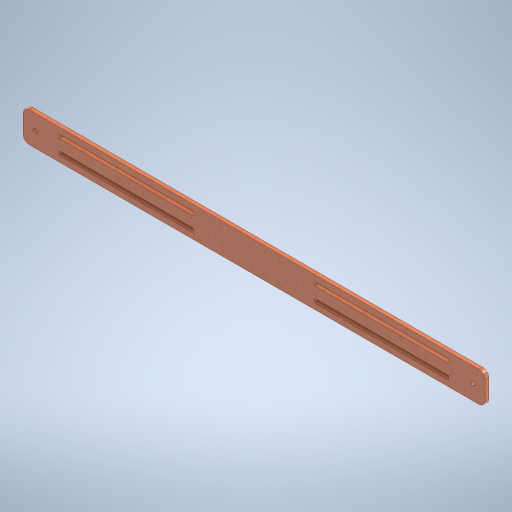
# Autodesk Inventor part: Pared
Saved by Autodesk Inventor 2024 (Build 280153000, 153)
## iProperties
Created: 2023-11-01
Part Number: Pared
Material: Generic
Document SubType Name: Modeling
Designer: fredy
Density: 1 g/cm^3
Appearance: Walnut - Natural Polished
Author: fredy
Autodesk Inventor part; units mm, degrees
ref_plane "YZ Plane" through (0, 0, 0) normal (1, 0, 0) x (0, 1, 0)
ref_plane "XZ Plane" through (0, 0, 0) normal (0, 1, 0) x (-1, 0, 0)
ref_plane "XY Plane" through (0, 0, 0) normal (0, 0, 1) x (1, 0, 0)
sketch "Sketch1" plane through (0, 0, 0) normal (0, 0, 1) x (1, 0, 0)
  line L0 (0, 0) -> (380, 0)
  line L1 (0, 0) -> (0, 25)
  line L2 (0, 25) -> (380, 25)
  line L3 (380, 25) -> (380, 0)
  dimension "d0" = 380
  dimension "d1" = 25
  constraints: 8 end point, 2 horizontal, 2 vertical, 1 coincident
  measures "d0" distance of L1.end L2.end
  measures "d1" distance of L0.start L1.end
extrude "Extrusion1" add sketch "Sketch1" along normal blind 3
fillet "Fillet1" radius 5 4 edges at (380, 25, 1.5) (380, 0, 1.5) (0, 25, 1.5) (0, 0, 1.5)
sketch "Sketch2" plane through (0, 0, 3) normal (0, 0, 1) x (1, 0, 0)
  line L0 (30, 16.9) -> (140, 16.9)
  line L1 (140, 16.9) -> (140, 20)
  line L2 (140, 20) -> (30, 20)
  line L3 (30, 20) -> (30, 16.9)
  line L4 (375, 25) -> (5, 25) projected
  line L5 (0, 20) -> (0, 5) projected
  line L6 (380, 5) -> (380, 20) projected
  line L7 (0, 20) -> (0, 5) projected
  line L8 (0, 12.5) -> (380, 12.5)
  line L9 (30, 8.1) -> (140, 8.1)
  line L10 (140, 8.1) -> (140, 5)
  line L11 (140, 5) -> (30, 5)
  line L12 (30, 5) -> (30, 8.1)
  line L13 (190, 25) -> (190, 0)
  line L14 (5, 0) -> (375, 0) projected
  line L15 (350, 16.9) -> (240, 16.9)
  line L16 (240, 16.9) -> (240, 20)
  line L17 (240, 20) -> (350, 20)
  line L18 (350, 20) -> (350, 16.9)
  line L19 (240, 8.1) -> (240, 5)
  line L20 (350, 5) -> (350, 8.1)
  line L21 (350, 8.1) -> (240, 8.1)
  line L22 (240, 5) -> (350, 5)
  point P0 (0, 0)
  point P1 (350, 18.45)
  point P2 (240, 18.45)
  point P3 (140, 18.45)
  dimension "d5" = 5
  dimension "d6" = 3.1
  dimension "d7" = 30
  dimension "d12" = 100
  constraints: 36 end point, 12 symmetric about line, 7 midpoint, 2 parallel, 1 horizontal, 1 perpendicular
  measures "d5" distance between parallel lines of L4 L2
  measures "d6" distance of L2.end L0.start
  measures "d7" distance between parallel lines of L5 L3
  measures "d12" distance of point (240, 18.45) point (140, 18.45)
extrude "Extrusion2" cut sketch "Sketch2" against normal up to surface (3 mm away)
sketch "Sketch3" plane through (0, 0, 3) normal (0, 0, 1) x (1, 0, 0)
  line L0 (0, 20) -> (0, 5) projected
  line L1 (0, 12.5) -> (20.3582, 12.5)
  line L2 (375, 25) -> (5, 25) projected
  line L3 (10, 25) -> (10, 0)
  line L4 (190, 25) -> (190, 0) construction
  line L5 (5, 0) -> (375, 0) construction
  point P0 (0, 0)
  point P1 (10, 12.5)
  point P2 (370, 12.5)
  dimension "d13" = 10
  constraints: 6 end point, 4 midpoint, 2 point on line, 2 vertical, 1 horizontal, 1 symmetric about line
  measures "d13" distance between parallel lines of L0 L3
hole "Hole1" at (10, 12.5, 3) at (370, 12.5, 3) direction (0, 0, -1) diameter 3.375 end through all
body "Solid1"
